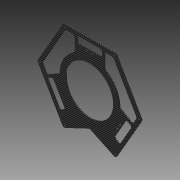
# Autodesk Inventor part: Bottom Plate
Saved by Autodesk Inventor 2015 (Build 190159000, 159)
## iProperties
Created: 2016-10-01
Part Number: Bottom Plate
Material: Generic
Document SubType Name: Modeling
Designer: James Yelland
Density: 1 g/cm^3
Appearance: Default
Author: James Yelland
Autodesk Inventor part; units mm, degrees
ref_plane "YZ Plane" through (0, 0, 0) normal (1, 0, 0) x (0, 1, 0)
ref_plane "XZ Plane" through (0, 0, 0) normal (0, 1, 0) x (-1, 0, 0)
ref_plane "XY Plane" through (0, 0, 0) normal (0, 0, 1) x (1, 0, 0)
sketch "Sketch1" plane through (0, 0, 0) normal (0, 1, 0) x (-1, 0, 0)
  line L0 (72.6878, -41.9663) -> (62.1878, -60.1529)
  line L1 (72.6878, -41.9663) -> (83.1878, -23.7798)
  line L2 (81.7237, -18.3157) -> (77.3936, -15.8157)
  line L3 (71.9295, -17.2797) -> (50.9295, -53.6529)
  line L4 (52.3936, -59.117) -> (56.7237, -61.617)
  arc A0 (56.7237, -61.617) -> (62.1878, -60.1529) centre (58.7237, -58.1529) ccw
  arc A1 (50.9295, -53.6529) -> (52.3936, -59.117) centre (54.3936, -55.6529) ccw
  arc A2 (77.3936, -15.8157) -> (71.9295, -17.2797) centre (75.3936, -19.2798) ccw
  arc A3 (83.1878, -23.7798) -> (81.7237, -18.3157) centre (79.7237, -21.7798) ccw
  line L5 (55.5994, -35.5644) -> (57.3314, -36.5644)
  line L6 (57.3314, -36.5644) -> (54.8314, -40.8945)
  line L7 (53.0994, -39.8945) -> (55.5994, -35.5644)
  line L8 (54.8314, -40.8945) -> (53.0994, -39.8945)
  line L9 (61.0994, -26.0381) -> (58.5994, -30.3683)
  line L10 (60.3314, -31.3683) -> (62.8314, -27.0381)
  line L11 (58.5994, -30.3683) -> (60.3314, -31.3683)
  line L12 (62.8314, -27.0381) -> (61.0994, -26.0381)
  line L13 (0, 83.9327) -> (21, 83.9327)
  line L14 (0, 83.9327) -> (-21, 83.9327)
  line L15 (-25, 79.9327) -> (-25, 74.9327)
  line L16 (-21, 70.9327) -> (20.9998, 70.9327)
  line L17 (25, 74.9327) -> (25, 79.9327)
  arc A4 (25, 79.9327) -> (21, 83.9327) centre (21, 79.9327) ccw
  arc A5 (20.9998, 70.9327) -> (25, 74.9327) centre (21, 74.9327) ccw
  arc A6 (-25, 74.9327) -> (-21, 70.9327) centre (-21, 74.9327) ccw
  arc A7 (-21, 83.9327) -> (-25, 79.9327) centre (-21, 79.9327) ccw
  line L18 (3, 65.9327) -> (3, 67.9327)
  line L19 (8, 65.9327) -> (3, 65.9327)
  line L20 (8, 67.9327) -> (8, 65.9327)
  line L21 (3, 67.9327) -> (8, 67.9327)
  line L22 (-8, 67.9327) -> (-8, 65.9327)
  line L23 (-8, 65.9327) -> (-3, 65.9327)
  line L24 (-3, 65.9327) -> (-3, 67.9327)
  line L25 (-3, 67.9327) -> (-8, 67.9327)
  line L26 (-72.6878, -41.9663) -> (-83.1878, -23.7798)
  line L27 (-72.6878, -41.9663) -> (-62.1878, -60.1529)
  line L28 (-56.7237, -61.617) -> (-52.3936, -59.117)
  line L29 (-50.9295, -53.6529) -> (-71.9294, -17.28)
  line L30 (-77.3936, -15.8157) -> (-81.7237, -18.3157)
  arc A8 (-81.7237, -18.3157) -> (-83.1878, -23.7798) centre (-79.7237, -21.7798) ccw
  arc A9 (-71.9294, -17.28) -> (-77.3936, -15.8157) centre (-75.3936, -19.2798) ccw
  arc A10 (-52.3936, -59.117) -> (-50.9295, -53.6529) centre (-54.3936, -55.6529) ccw
  arc A11 (-62.1878, -60.1529) -> (-56.7237, -61.617) centre (-58.7237, -58.1529) ccw
  line L31 (-58.5994, -30.3683) -> (-60.3314, -31.3683)
  line L32 (-61.0994, -26.0381) -> (-58.5994, -30.3683)
  line L33 (-62.8314, -27.0381) -> (-61.0994, -26.0381)
  line L34 (-60.3314, -31.3683) -> (-62.8314, -27.0381)
  line L35 (-54.8314, -40.8945) -> (-53.0994, -39.8945)
  line L36 (-53.0994, -39.8945) -> (-55.5994, -35.5644)
  line L37 (-55.5994, -35.5644) -> (-57.3314, -36.5644)
  line L38 (-57.3314, -36.5644) -> (-54.8314, -40.8945)
  line L39 (103.5566, -2.5) -> (54.8095, -86.9325)
  line L40 (-54.8095, -86.9325) -> (-103.5566, -2.5)
  line L41 (-103.5566, 2.5) -> (-53.9434, 88.4327)
  line L42 (-49.6132, 90.9327) -> (49.6132, 90.9327)
  line L43 (53.9434, 88.4327) -> (103.5566, 2.5)
  line L44 (2.1497, -66.9563) -> (48.3297, -88.9468)
  line L45 (-2.1497, -66.9563) -> (-48.3297, -88.9468)
  arc A12 (48.3297, -88.9468) -> (54.8095, -86.9325) centre (50.4794, -84.4325) ccw
  arc A13 (2.1497, -66.9563) -> (-2.1497, -66.9563) centre (0, -71.4706) ccw
  arc A14 (-54.8095, -86.9325) -> (-48.3297, -88.9468) centre (-50.4794, -84.4325) ccw
  arc A15 (-103.5566, 2.5) -> (-103.5566, -2.5) centre (-99.2265, 0) ccw
  arc A16 (-49.6132, 90.9327) -> (-53.9434, 88.4327) centre (-49.6132, 85.9327) ccw
  arc A17 (53.9434, 88.4327) -> (49.6132, 90.9327) centre (49.6132, 85.9327) ccw
  arc A18 (103.5566, -2.5) -> (103.5566, 2.5) centre (99.2265, 0) ccw
  circle A19 centre (49.6132, 85.9327) radius 1.6
  circle A20 centre (-49.6132, 85.9327) radius 1.6
  circle A21 centre (-99.2265, 0) radius 1.6
  circle A22 centre (99.2265, 0) radius 1.6
  line L46 (48.9434, 79.7724) -> (93.5566, 2.5)
  line L47 (-35, 82.2724) -> (-44.6132, 82.2724)
  line L48 (35, 82.2724) -> (44.6132, 82.2724)
  arc A23 (35, 82.2724) -> (30, 77.2724) centre (35, 77.2724) ccw
  arc A24 (-30, 77.2724) -> (-35, 82.2724) centre (-35, 77.2724) ccw
  arc A25 (48.9434, 79.7724) -> (44.6132, 82.2724) centre (44.6132, 77.2724) ccw
  line L49 (-93.5566, 2.5) -> (-48.9434, 79.7724)
  line L50 (-88.75, -10.8253) -> (-93.5566, -2.5)
  arc A26 (-88.75, -10.8253) -> (-81.9199, -12.6554) centre (-84.4199, -8.3253) ccw
  arc A27 (-93.5566, 2.5) -> (-93.5566, -2.5) centre (-89.2265, 0) ccw
  line L51 (88.75, -10.8253) -> (93.5566, -2.5)
  arc A28 (81.9199, -12.6554) -> (88.75, -10.8253) centre (84.4199, -8.3253) ccw
  arc A29 (-44.6132, 82.2724) -> (-48.9434, 79.7724) centre (-44.6132, 77.2724) ccw
  arc A30 (93.5566, -2.5) -> (93.5566, 2.5) centre (89.2265, 0) ccw
  line L52 (81.9199, -12.6554) -> (61.4758, -0.8521)
  line L53 (30, 77.2724) -> (30, 53.6656)
  line L54 (-30, 77.2724) -> (-30, 53.6656)
  line L55 (-81.9199, -12.6554) -> (-61.4758, -0.8521)
  circle A31 centre (0, 0) radius 47.5
  arc A32 (59.977, 1.6629) -> (31.4286, 51.1101) centre (0, 0) ccw
  arc A33 (-31.4286, 51.1101) -> (-59.977, 1.6629) centre (0, 0) ccw
  arc A34 (59.977, 1.6629) -> (61.4758, -0.8521) centre (62.9758, 1.746) ccw
  arc A35 (30, 53.6656) -> (31.4286, 51.1101) centre (33, 53.6656) ccw
  arc A36 (-31.4286, 51.1101) -> (-30, 53.6656) centre (-33, 53.6656) ccw
  arc A37 (-61.4758, -0.8521) -> (-59.977, 1.6629) centre (-62.9758, 1.746) ccw
  circle A38 centre (50.4794, -84.4325) radius 1.6
  circle A39 centre (-50.4794, -84.4325) radius 1.6
  circle A40 centre (0, 0) radius 53.75
  line L56 (0, -53.75) -> (-1.5, -53.75)
  line L57 (0, -53.75) -> (1.5, -53.75)
  line L58 (1.5, -53.75) -> (1.5, -56.75)
  line L59 (1.5, -56.75) -> (4.5, -56.75)
  line L60 (4.5, -56.75) -> (4.5, -50.75)
  line L61 (4.5, -50.75) -> (1.5, -50.75)
  line L62 (1.5, -50.75) -> (1.5, -53.75)
  line L63 (-1.5, -53.75) -> (-1.5, -56.75)
  line L64 (-1.5, -56.75) -> (-4.5, -56.75)
  line L65 (-1.5, -53.75) -> (-1.5, -53.75)
  line L66 (-1.5, -53.75) -> (-1.5, -50.75)
  line L67 (-1.5, -53.75) -> (1.5, -53.75) construction
  line L68 (-1.5, -50.75) -> (-4.5, -50.75)
  line L69 (-4.5, -56.75) -> (-4.5, -50.75)
  line L70 (15.3604, -51.5303) -> (16.1369, -54.4281)
  line L71 (16.1369, -54.4281) -> (19.0346, -53.6516)
  line L72 (19.0346, -53.6516) -> (17.4817, -47.856)
  line L73 (17.4817, -47.856) -> (14.584, -48.6325)
  line L74 (14.584, -48.6325) -> (15.3604, -51.5303)
  line L75 (12.4626, -52.3067) -> (13.2391, -55.2045)
  line L76 (13.2391, -55.2045) -> (10.3413, -55.981)
  line L77 (12.4626, -52.3067) -> (11.6862, -49.409)
  line L78 (11.6862, -49.409) -> (8.7884, -50.1854)
  line L79 (10.3413, -55.981) -> (8.7884, -50.1854)
  line L80 (28.174, -45.7989) -> (29.674, -48.3969)
  line L81 (29.674, -48.3969) -> (32.2721, -46.8969)
  line L82 (32.2721, -46.8969) -> (29.2721, -41.7008)
  line L83 (29.2721, -41.7008) -> (26.674, -43.2008)
  line L84 (26.674, -43.2008) -> (28.174, -45.7989)
  line L85 (25.576, -47.2989) -> (27.076, -49.8969)
  line L86 (27.076, -49.8969) -> (24.4779, -51.3969)
  line L87 (25.576, -47.2989) -> (24.076, -44.7008)
  line L88 (24.076, -44.7008) -> (21.4779, -46.2008)
  line L89 (24.4779, -51.3969) -> (21.4779, -46.2008)
  line L90 (39.0676, -36.9463) -> (41.189, -39.0676)
  line L91 (41.189, -39.0676) -> (43.3103, -36.9463)
  line L92 (43.3103, -36.9463) -> (39.0676, -32.7037)
  line L93 (39.0676, -32.7037) -> (36.9463, -34.825)
  line L94 (36.9463, -34.825) -> (39.0676, -36.9463)
  line L95 (36.9463, -39.0676) -> (39.0676, -41.189)
  line L96 (39.0676, -41.189) -> (36.9463, -43.3103)
  line L97 (36.9463, -39.0676) -> (34.825, -36.9463)
  line L98 (34.825, -36.9463) -> (32.7037, -39.0676)
  line L99 (36.9463, -43.3103) -> (32.7037, -39.0676)
  line L100 (47.2989, -25.576) -> (49.8969, -27.076)
  line L101 (49.8969, -27.076) -> (51.3969, -24.4779)
  line L102 (51.3969, -24.4779) -> (46.2008, -21.4779)
  line L103 (46.2008, -21.4779) -> (44.7008, -24.076)
  line L104 (44.7008, -24.076) -> (47.2989, -25.576)
  line L105 (45.7989, -28.174) -> (48.3969, -29.674)
  line L106 (48.3969, -29.674) -> (46.8969, -32.2721)
  line L107 (45.7989, -28.174) -> (43.2008, -26.674)
  line L108 (43.2008, -26.674) -> (41.7008, -29.2721)
  line L109 (46.8969, -32.2721) -> (41.7008, -29.2721)
  line L110 (52.3067, -12.4626) -> (55.2045, -13.2391)
  line L111 (55.2045, -13.2391) -> (55.981, -10.3413)
  line L112 (55.981, -10.3413) -> (50.1854, -8.7884)
  line L113 (50.1854, -8.7884) -> (49.409, -11.6862)
  line L114 (49.409, -11.6862) -> (52.3067, -12.4626)
  line L115 (51.5303, -15.3604) -> (54.4281, -16.1369)
  line L116 (54.4281, -16.1369) -> (53.6516, -19.0346)
  line L117 (51.5303, -15.3604) -> (48.6325, -14.584)
  line L118 (48.6325, -14.584) -> (47.856, -17.4817)
  line L119 (53.6516, -19.0346) -> (47.856, -17.4817)
  line L120 (53.75, 1.5) -> (56.75, 1.5)
  line L121 (56.75, 1.5) -> (56.75, 4.5)
  line L122 (56.75, 4.5) -> (50.75, 4.5)
  line L123 (50.75, 4.5) -> (50.75, 1.5)
  line L124 (50.75, 1.5) -> (53.75, 1.5)
  line L125 (53.75, -1.5) -> (56.75, -1.5)
  line L126 (56.75, -1.5) -> (56.75, -4.5)
  line L127 (53.75, -1.5) -> (50.75, -1.5)
  line L128 (50.75, -1.5) -> (50.75, -4.5)
  line L129 (56.75, -4.5) -> (50.75, -4.5)
  line L130 (51.5303, 15.3604) -> (54.4281, 16.1369)
  line L131 (54.4281, 16.1369) -> (53.6516, 19.0346)
  line L132 (53.6516, 19.0346) -> (47.856, 17.4817)
  line L133 (47.856, 17.4817) -> (48.6325, 14.584)
  line L134 (48.6325, 14.584) -> (51.5303, 15.3604)
  line L135 (52.3067, 12.4626) -> (55.2045, 13.2391)
  line L136 (55.2045, 13.2391) -> (55.981, 10.3413)
  line L137 (52.3067, 12.4626) -> (49.409, 11.6862)
  line L138 (49.409, 11.6862) -> (50.1854, 8.7884)
  line L139 (55.981, 10.3413) -> (50.1854, 8.7884)
  line L140 (45.7989, 28.174) -> (48.3969, 29.674)
  line L141 (48.3969, 29.674) -> (46.8969, 32.2721)
  line L142 (46.8969, 32.2721) -> (41.7008, 29.2721)
  line L143 (41.7008, 29.2721) -> (43.2008, 26.674)
  line L144 (43.2008, 26.674) -> (45.7989, 28.174)
  line L145 (47.2989, 25.576) -> (49.8969, 27.076)
  line L146 (49.8969, 27.076) -> (51.3969, 24.4779)
  line L147 (47.2989, 25.576) -> (44.7008, 24.076)
  line L148 (44.7008, 24.076) -> (46.2008, 21.4779)
  line L149 (51.3969, 24.4779) -> (46.2008, 21.4779)
  line L150 (36.9463, 39.0676) -> (39.0676, 41.189)
  line L151 (39.0676, 41.189) -> (36.9463, 43.3103)
  line L152 (36.9463, 43.3103) -> (32.7037, 39.0676)
  line L153 (32.7037, 39.0676) -> (34.825, 36.9463)
  line L154 (34.825, 36.9463) -> (36.9463, 39.0676)
  line L155 (39.0676, 36.9463) -> (41.189, 39.0676)
  line L156 (41.189, 39.0676) -> (43.3103, 36.9463)
  line L157 (39.0676, 36.9463) -> (36.9463, 34.825)
  line L158 (36.9463, 34.825) -> (39.0676, 32.7037)
  line L159 (43.3103, 36.9463) -> (39.0676, 32.7037)
  line L160 (25.576, 47.2989) -> (27.076, 49.8969)
  line L161 (27.076, 49.8969) -> (24.4779, 51.3969)
  line L162 (24.4779, 51.3969) -> (21.4779, 46.2008)
  line L163 (21.4779, 46.2008) -> (24.076, 44.7008)
  line L164 (24.076, 44.7008) -> (25.576, 47.2989)
  line L165 (28.174, 45.7989) -> (29.674, 48.3969)
  line L166 (29.674, 48.3969) -> (32.2721, 46.8969)
  line L167 (28.174, 45.7989) -> (26.674, 43.2008)
  line L168 (26.674, 43.2008) -> (29.2721, 41.7008)
  line L169 (32.2721, 46.8969) -> (29.2721, 41.7008)
  line L170 (12.4626, 52.3067) -> (13.2391, 55.2045)
  line L171 (13.2391, 55.2045) -> (10.3413, 55.981)
  line L172 (10.3413, 55.981) -> (8.7884, 50.1854)
  line L173 (8.7884, 50.1854) -> (11.6862, 49.409)
  line L174 (11.6862, 49.409) -> (12.4626, 52.3067)
  line L175 (15.3604, 51.5303) -> (16.1369, 54.4281)
  line L176 (16.1369, 54.4281) -> (19.0346, 53.6516)
  line L177 (15.3604, 51.5303) -> (14.584, 48.6325)
  line L178 (14.584, 48.6325) -> (17.4817, 47.856)
  line L179 (19.0346, 53.6516) -> (17.4817, 47.856)
  line L180 (-1.5, 53.75) -> (-1.5, 56.75)
  line L181 (-1.5, 56.75) -> (-4.5, 56.75)
  line L182 (-4.5, 56.75) -> (-4.5, 50.75)
  line L183 (-4.5, 50.75) -> (-1.5, 50.75)
  line L184 (-1.5, 50.75) -> (-1.5, 53.75)
  line L185 (1.5, 53.75) -> (1.5, 56.75)
  line L186 (1.5, 56.75) -> (4.5, 56.75)
  line L187 (1.5, 53.75) -> (1.5, 50.75)
  line L188 (1.5, 50.75) -> (4.5, 50.75)
  line L189 (4.5, 56.75) -> (4.5, 50.75)
  line L190 (-15.3604, 51.5303) -> (-16.1369, 54.4281)
  line L191 (-16.1369, 54.4281) -> (-19.0346, 53.6516)
  line L192 (-19.0346, 53.6516) -> (-17.4817, 47.856)
  line L193 (-17.4817, 47.856) -> (-14.584, 48.6325)
  line L194 (-14.584, 48.6325) -> (-15.3604, 51.5303)
  line L195 (-12.4626, 52.3067) -> (-13.2391, 55.2045)
  line L196 (-13.2391, 55.2045) -> (-10.3413, 55.981)
  line L197 (-12.4626, 52.3067) -> (-11.6862, 49.409)
  line L198 (-11.6862, 49.409) -> (-8.7884, 50.1854)
  line L199 (-10.3413, 55.981) -> (-8.7884, 50.1854)
  line L200 (-28.174, 45.7989) -> (-29.674, 48.3969)
  line L201 (-29.674, 48.3969) -> (-32.2721, 46.8969)
  line L202 (-32.2721, 46.8969) -> (-29.2721, 41.7008)
  line L203 (-29.2721, 41.7008) -> (-26.674, 43.2008)
  line L204 (-26.674, 43.2008) -> (-28.174, 45.7989)
  line L205 (-25.576, 47.2989) -> (-27.076, 49.8969)
  line L206 (-27.076, 49.8969) -> (-24.4779, 51.3969)
  line L207 (-25.576, 47.2989) -> (-24.076, 44.7008)
  line L208 (-24.076, 44.7008) -> (-21.4779, 46.2008)
  line L209 (-24.4779, 51.3969) -> (-21.4779, 46.2008)
  line L210 (-39.0676, 36.9463) -> (-41.189, 39.0676)
  line L211 (-41.189, 39.0676) -> (-43.3103, 36.9463)
  line L212 (-43.3103, 36.9463) -> (-39.0676, 32.7037)
  line L213 (-39.0676, 32.7037) -> (-36.9463, 34.825)
  line L214 (-36.9463, 34.825) -> (-39.0676, 36.9463)
  line L215 (-36.9463, 39.0676) -> (-39.0676, 41.189)
  line L216 (-39.0676, 41.189) -> (-36.9463, 43.3103)
  line L217 (-36.9463, 39.0676) -> (-34.825, 36.9463)
  line L218 (-34.825, 36.9463) -> (-32.7037, 39.0676)
  line L219 (-36.9463, 43.3103) -> (-32.7037, 39.0676)
  line L220 (-47.2989, 25.576) -> (-49.8969, 27.076)
  line L221 (-49.8969, 27.076) -> (-51.3969, 24.4779)
  line L222 (-51.3969, 24.4779) -> (-46.2008, 21.4779)
  line L223 (-46.2008, 21.4779) -> (-44.7008, 24.076)
  line L224 (-44.7008, 24.076) -> (-47.2989, 25.576)
  line L225 (-45.7989, 28.174) -> (-48.3969, 29.674)
  line L226 (-48.3969, 29.674) -> (-46.8969, 32.2721)
  line L227 (-45.7989, 28.174) -> (-43.2008, 26.674)
  line L228 (-43.2008, 26.674) -> (-41.7008, 29.2721)
  line L229 (-46.8969, 32.2721) -> (-41.7008, 29.2721)
  line L230 (-52.3067, 12.4626) -> (-55.2045, 13.2391)
  line L231 (-55.2045, 13.2391) -> (-55.981, 10.3413)
  line L232 (-55.981, 10.3413) -> (-50.1854, 8.7884)
  line L233 (-50.1854, 8.7884) -> (-49.409, 11.6862)
  line L234 (-49.409, 11.6862) -> (-52.3067, 12.4626)
  line L235 (-51.5303, 15.3604) -> (-54.4281, 16.1369)
  line L236 (-54.4281, 16.1369) -> (-53.6516, 19.0346)
  line L237 (-51.5303, 15.3604) -> (-48.6325, 14.584)
  line L238 (-48.6325, 14.584) -> (-47.856, 17.4817)
  line L239 (-53.6516, 19.0346) -> (-47.856, 17.4817)
  line L240 (-53.75, -1.5) -> (-56.75, -1.5)
  line L241 (-56.75, -1.5) -> (-56.75, -4.5)
  line L242 (-56.75, -4.5) -> (-50.75, -4.5)
  line L243 (-50.75, -4.5) -> (-50.75, -1.5)
  line L244 (-50.75, -1.5) -> (-53.75, -1.5)
  line L245 (-53.75, 1.5) -> (-56.75, 1.5)
  line L246 (-56.75, 1.5) -> (-56.75, 4.5)
  line L247 (-53.75, 1.5) -> (-50.75, 1.5)
  line L248 (-50.75, 1.5) -> (-50.75, 4.5)
  line L249 (-56.75, 4.5) -> (-50.75, 4.5)
  line L250 (-51.5303, -15.3604) -> (-54.4281, -16.1369)
  line L251 (-54.4281, -16.1369) -> (-53.6516, -19.0346)
  line L252 (-53.6516, -19.0346) -> (-47.856, -17.4817)
  line L253 (-47.856, -17.4817) -> (-48.6325, -14.584)
  line L254 (-48.6325, -14.584) -> (-51.5303, -15.3604)
  line L255 (-52.3067, -12.4626) -> (-55.2045, -13.2391)
  line L256 (-55.2045, -13.2391) -> (-55.981, -10.3413)
  line L257 (-52.3067, -12.4626) -> (-49.409, -11.6862)
  line L258 (-49.409, -11.6862) -> (-50.1854, -8.7884)
  line L259 (-55.981, -10.3413) -> (-50.1854, -8.7884)
  line L260 (-45.7989, -28.174) -> (-48.3969, -29.674)
  line L261 (-48.3969, -29.674) -> (-46.8969, -32.2721)
  line L262 (-46.8969, -32.2721) -> (-41.7008, -29.2721)
  line L263 (-41.7008, -29.2721) -> (-43.2008, -26.674)
  line L264 (-43.2008, -26.674) -> (-45.7989, -28.174)
  line L265 (-47.2989, -25.576) -> (-49.8969, -27.076)
  line L266 (-49.8969, -27.076) -> (-51.3969, -24.4779)
  line L267 (-47.2989, -25.576) -> (-44.7008, -24.076)
  line L268 (-44.7008, -24.076) -> (-46.2008, -21.4779)
  line L269 (-51.3969, -24.4779) -> (-46.2008, -21.4779)
  line L270 (-36.9463, -39.0676) -> (-39.0676, -41.189)
  line L271 (-39.0676, -41.189) -> (-36.9463, -43.3103)
  line L272 (-36.9463, -43.3103) -> (-32.7037, -39.0676)
  line L273 (-32.7037, -39.0676) -> (-34.825, -36.9463)
  line L274 (-34.825, -36.9463) -> (-36.9463, -39.0676)
  line L275 (-39.0676, -36.9463) -> (-41.189, -39.0676)
  line L276 (-41.189, -39.0676) -> (-43.3103, -36.9463)
  line L277 (-39.0676, -36.9463) -> (-36.9463, -34.825)
  line L278 (-36.9463, -34.825) -> (-39.0676, -32.7037)
  line L279 (-43.3103, -36.9463) -> (-39.0676, -32.7037)
  line L280 (-25.576, -47.2989) -> (-27.076, -49.8969)
  line L281 (-27.076, -49.8969) -> (-24.4779, -51.3969)
  line L282 (-24.4779, -51.3969) -> (-21.4779, -46.2008)
  line L283 (-21.4779, -46.2008) -> (-24.076, -44.7008)
  line L284 (-24.076, -44.7008) -> (-25.576, -47.2989)
  line L285 (-28.174, -45.7989) -> (-29.674, -48.3969)
  line L286 (-29.674, -48.3969) -> (-32.2721, -46.8969)
  line L287 (-28.174, -45.7989) -> (-26.674, -43.2008)
  line L288 (-26.674, -43.2008) -> (-29.2721, -41.7008)
  line L289 (-32.2721, -46.8969) -> (-29.2721, -41.7008)
  line L290 (-12.4626, -52.3067) -> (-13.2391, -55.2045)
  line L291 (-13.2391, -55.2045) -> (-10.3413, -55.981)
  line L292 (-10.3413, -55.981) -> (-8.7884, -50.1854)
  line L293 (-8.7884, -50.1854) -> (-11.6862, -49.409)
  line L294 (-11.6862, -49.409) -> (-12.4626, -52.3067)
  line L295 (-15.3604, -51.5303) -> (-16.1369, -54.4281)
  line L296 (-16.1369, -54.4281) -> (-19.0346, -53.6516)
  line L297 (-15.3604, -51.5303) -> (-14.584, -48.6325)
  line L298 (-14.584, -48.6325) -> (-17.4817, -47.856)
  line L299 (-19.0346, -53.6516) -> (-17.4817, -47.856)
  point P0 (60.1878, -63.617)
  point P1 (85.1878, -20.3157)
  point P2 (73.9295, -13.8157)
  point P3 (48.9295, -57.117)
  point P4 (25, 83.9327)
  point P5 (-25, 83.9327)
  point P6 (-25, 70.9327)
  point P7 (25, 70.9327)
  point P8 (-85.1878, -20.3157)
  point P9 (-60.1878, -63.617)
  point P10 (-48.9295, -57.117)
  point P11 (-73.9295, -13.8157)
  point P12 (105, 0)
  point P13 (52.5, -90.9327)
  point P14 (-105, 0)
  point P15 (-52.5, 90.9327)
  point P16 (52.5, 90.9327)
  point P17 (-86.25, -15.1554)
  point P18 (60, 0)
  point P19 (30, 51.9615)
  point P20 (-30, 51.9615)
  point P21 (-60, 0)
  dimension "d11" = 360
  dimension "d30" = 360
  dimension "d32" = 5
  dimension "d53" = 3
  dimension "d59" = 3.2
  dimension "d60" = 3.2
  dimension "d61" = 107.5
  dimension "d80" = 360
  constraints: 600 end point, 70 point on circle, 63 point on line, 41 centre point, 12 tangent, 9 coincident, 6 perpendicular, 4 equal radius, 4 horizontal, 4 vertical, 505 other
  measures "d32" radius of A29
  measures "d53" radius of A34
  measures "d59" diameter of A38
  measures "d60" diameter of A39
  measures "d61" diameter of A40
extrude "Extrusion1" add sketch "Sketch1" along normal blind 2 contours L39 A12 L44 A13 L45 A14 L40 A15 L41 A16 L42 A17 L43 A18 | A40 L127 L128 L129 L112 L113 L114 L117 L118 L119 L102 L103 L104 L107 L108 L109 L92 L93 L94 L97 L98 L99 L82 L83 L84 L87 L88 L89 L72 L73 L74 L77 L78 L79 L60 L61 L62 L66 L68 L69 L292 L293 L294 L297 L298 L299 L282 L283 L284 L287 L288 L289 L272 L273 L274 L277 L278 L279 L262 L263 L264 L267 L268 L269 L252 L253 L254 L257 L258 L259 L242 L243 L244 L247 L248 L249 L232 L233 L234 L237 L238 L239 L222 L223 L224 L227 L228 L229 L212 L213 L214 L217 L218 L219 L202 L203 L204 L207 L208 L209 L192 L193 L194 L197 L198 L199 L182 L183 L184 L187 L188 L189 L172 L173 L174 L177 L178 L179 L162 L163 L164 L167 L168 L169 L152 L153 L154 L157 L158 L159 L142 L143 L144 L147 L148 L149 L132 L133 L134 L137 L138 L139 L122 L123 L124 | L124 L123 L122 A40 | A40 L122 L121 L120 L124 | L127 L125 L126 L129 A40 | A40 L129 L128 L127 | L139 L138 L137 A40 | A40 L137 L135 L136 L139 | L112 L111 L110 L114 A40 | A40 L114 L113 L112 | L134 L133 L132 A40 | A40 L132 L131 L130 L134 | L117 L115 L116 L119 A40 | A40 L119 L118 L117 | L149 L148 L147 A40 | A40 L147 L145 L146 L149 | L102 L101 L100 L104 A40 | A40 L104 L103 L102 | L144 L143 L142 A40 | A40 L142 L141 L140 L144 | L107 L105 L106 L109 A40 | A40 L109 L108 L107 | L159 L158 L157 A40 | A40 L157 L155 L156 L159 | L92 L91 L90 L94 A40 | A40 L94 L93 L92 | L154 L153 L152 A40 | A40 L152 L151 L150 L154 | L97 L95 L96 L99 A40 | A40 L99 L98 L97 | L169 L168 L167 A40 | A40 L167 L165 L166 L169 | L82 L81 L80 L84 A40 | A40 L84 L83 L82 | L164 L163 L162 A40 | A40 L162 L161 L160 L164 | L87 L85 L86 L89 A40 | A40 L89 L88 L87 | L179 L178 L177 A40 | A40 L177 L175 L176 L179 | L72 L71 L70 L74 A40 | A40 L74 L73 L72 | L174 L173 L172 A40 | A40 L172 L171 L170 L174 | L77 L75 L76 L79 A40 | A40 L79 L78 L77 | L189 L188 L187 A40 | A40 L187 L185 L186 L189 | L60 L59 L58 L62 A40 | A40 L62 L61 L60 | L62 L57 A40 | L184 L183 L182 A40 | A40 L182 L181 L180 L184 | L56 L66 A40 | L66 L63 L64 L69 A40 | A40 L69 L68 L66 | L199 L198 L197 A40 | A40 L197 L195 L196 L199 | L292 L291 L290 L294 A40 | A40 L294 L293 L292 | L194 L193 L192 A40 | A40 L192 L191 L190 L194 | L297 L295 L296 L299 A40 | A40 L299 L298 L297 | L209 L208 L207 A40 | A40 L207 L205 L206 L209 | L282 L281 L280 L284 A40 | A40 L284 L283 L282 | L204 L203 L202 A40 | A40 L202 L201 L200 L204 | L287 L285 L286 L289 A40 | A40 L289 L288 L287 | L219 L218 L217 A40 | A40 L217 L215 L216 L219 | L272 L271 L270 L274 A40 | A40 L274 L273 L272 | L214 L213 L212 A40 | A40 L212 L211 L210 L214 | L277 L275 L276 L279 A40 | A40 L279 L278 L277 | L229 L228 L227 A40 | A40 L227 L225 L226 L229 | L262 L261 L260 L264 A40 | A40 L264 L263 L262 | L224 L223 L222 A40 | A40 L222 L221 L220 L224 | L267 L265 L266 L269 A40 | A40 L269 L268 L267 | L239 L238 L237 A40 | A40 L237 L235 L236 L239 | L252 L251 L250 L254 A40 | A40 L254 L253 L252 | L234 L233 L232 A40 | A40 L232 L231 L230 L234 | L257 L255 L256 L259 A40 | A40 L259 L258 L257 | L249 L248 L247 A40 | A40 L247 L245 L246 L249 | L242 L241 L240 L244 A40 | A40 L244 L243 L242
body "Solid1"
